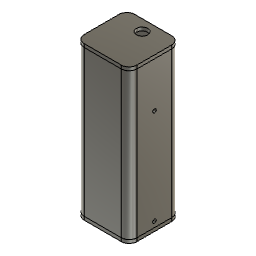
Blinds Device v2 (Autodesk Fusion 360 design; units mm, degrees)
Autodesk Fusion 360 part; units mm, degrees
sketch "Sketch1" plane through (0, 0, 0) normal (0, 0, 1) x (1, 0, 0)
  line L0 (0, 0) -> (39, 0)
  line L1 (0, 0) -> (0, 39)
  line L2 (0, 39) -> (39, 39)
  line L3 (39, 39) -> (39, 0)
  line L4 (39, 0) -> (0, 0)
  line L5 (0, 0) -> (0, 39)
  line L6 (0, 0) -> (3, 0)
  line L7 (39, 39) -> (36, 39)
  line L8 (39, 39) -> (42, 39)
  line L9 (0, 0) -> (-3, 0)
  line L10 (42, 39) -> (42, 42)
  line L11 (-3, 0) -> (-3, -3)
  line L12 (-3, -3) -> (42, -3)
  line L13 (42, -3) -> (42, 42)
  line L14 (42, 42) -> (-3, 42)
  line L15 (-3, 42) -> (-3, -3)
  dimension "d2" = 39
  dimension "d7" = 3
  dimension "d8" = 3
  dimension "d9" = 3
  dimension "d10" = 3
  constraint coincident L0.start L1.start
  constraint horizontal L0
  constraint vertical L1
  constraint horizontal L2
  constraint vertical L3
  constraint horizontal L4
  constraint vertical L5
  constraint perpendicular L1 L6
  constraint perpendicular L3 L7
  constraint perpendicular L3 L8
  constraint perpendicular L1 L9
  constraint perpendicular L8 L10
  constraint perpendicular L9 L11
  constraint horizontal L12
  constraint vertical L13
  constraint horizontal L14
  constraint vertical L15
  measures "d2" distance of L0.start L1.end
  measures "d7" distance of L2.end L8.end
  measures "d8" distance of L0.start L9.end
  measures "d9" distance of L8.end L10.end
  measures "d10" distance of L9.end L11.end
extrude "Extrude1" add sketch "Sketch1" along normal blind 130 contours L1 L2 L5 L7 L8 L9 L10 L13 L14 L15 | L0 L3 L4 L6 L8 L9 L11 L12 L13 L15 makes body 1
sketch "Sketch2" plane through (0, 0, 130) normal (0, 0, 1) x (-1, 0, 0)
  line L0 (-39, -39) -> (-39, 0)
  line L1 (-39, 0) -> (0, 0)
  line L2 (0, 0) -> (0, -39)
  line L3 (0, -39) -> (-39, -39)
  line L4 (3, -42) -> (3, 3)
  line L5 (3, 3) -> (-42, 3)
  line L6 (-42, 3) -> (-42, -42)
  line L7 (-42, -42) -> (3, -42)
  line L8 (3, -42) -> (-42, -42)
  line L9 (-42, -42) -> (-42, 3)
  line L10 (-42, 3) -> (3, 3)
  line L11 (3, 3) -> (3, -42)
  line L12 (-19.5, -42) -> (-19.5, -32)
  circle A0 centre (-19.5, -32) radius 5
  dimension "d13" = 10
  dimension "d14" = 10
  constraint horizontal L8
  constraint vertical L9
  constraint horizontal L10
  constraint vertical L11
  constraint coincident L5.end L6.start
  constraint coincident L4.start L7.end
  constraint midpoint L8 L12.start
  constraint perpendicular L8 L12
  constraint coincident L12.end A0.centre
  measures "d13" distance of L12.start L12.end
  measures "d14" diameter of A0
extrude "Extrude2" add sketch "Sketch2" along normal blind 3 separate body contours L0 L1 L2 L3 | L4 L5 L6 L7 L8 L9 L10 L11 makes body 2
extrude "Extrude3" cut 1 faces at (39, 26, 86.6667) along direction (1, 0, 0) blind 1 on bodies 1 bodies 1
extrude "Extrude4" cut 1 faces at (0, 13, 86.6667) along direction (-1, 0, 0) blind 1 on bodies 1 bodies 1
extrude "Extrude5" cut 1 faces at (-1, 13, 86.6667) along direction (-1, 0, 0) blind 1 on bodies 1 bodies 1
extrude "Extrude6" cut 1 faces at (40, 26, 86.6667) along direction (1, 0, 0) blind 1 on bodies 1 bodies 1
extrude "Extrude7" add 1 faces at (42, 12, 86.6667) along direction (1, 0, 0) blind 1 on bodies 1 bodies 1
extrude "Extrude8" add 1 faces at (-3, 27, 86.6667) along direction (-1, 0, 0) blind 1 on bodies 1 bodies 1
extrude "Extrude9" add 1 faces at (-3, 27, 132) along direction (-1, 0, 0) blind 1 on bodies 2 bodies 2
extrude "Extrude10" add 1 faces at (42, 12, 132) along direction (1, 0, 0) blind 1 on bodies 2 bodies 2
sketch "Sketch3" plane through (0, 0, 130) normal (0, 0, -1) x (1, 0, 0)
  circle A0 centre (19.5, -32) radius 5
  line L0 (43, 3) -> (-4, 3)
  line L1 (-4, 3) -> (-4, -42)
  line L2 (-4, -42) -> (43, -42)
  line L3 (43, -42) -> (43, 3)
  line L4 (43, 3) -> (40.8, 3)
  line L5 (40.8, 3) -> (40.8, -42)
  line L6 (19.5, -42) -> (19.5, 3)
  line L7 (43, -19.5) -> (-4, -19.5)
  line L8 (40.8, 3) -> (40.8, -0.2)
  line L9 (40.8, -0.2) -> (38.8, -0.2)
  line L10 (38.8, -0.2) -> (40.8, -0.2)
  line L11 (40.8, -0.2) -> (40.8, -10.2)
  line L12 (40.8, -10.2) -> (38.8, -10.2)
  line L13 (38.8, -10.2) -> (38.8, -0.2)
  line L14 (38.8, -28.8) -> (38.8, -38.8)
  line L15 (38.8, -38.8) -> (40.8, -38.8)
  line L16 (40.8, -28.8) -> (38.8, -28.8)
  line L17 (40.8, -38.8) -> (40.8, -28.8)
  line L18 (-1.8, -38.8) -> (-1.8, -28.8)
  line L19 (-1.8, -28.8) -> (0.2, -28.8)
  line L20 (0.2, -28.8) -> (0.2, -38.8)
  line L21 (0.2, -38.8) -> (-1.8, -38.8)
  line L22 (-1.8, -0.2) -> (-1.8, -10.2)
  line L23 (-1.8, -10.2) -> (0.2, -10.2)
  line L24 (-1.8, -0.2) -> (0.2, -0.2)
  line L25 (0.2, -10.2) -> (0.2, -0.2)
  dimension "d33" = 2.2
  dimension "d34" = 3.2
  dimension "d35" = 2
  dimension "d36" = 10
  constraint coincident L0.start L3.end
  constraint perpendicular L3 L4
  constraint coincident L2 L5.end
  constraint perpendicular L2 L5
  constraint midpoint L2 L6.start
  constraint midpoint L0 L6.end
  constraint midpoint L3 L7.start
  constraint midpoint L1 L7.end
  constraint perpendicular L4 L8
  constraint perpendicular L8 L9
  constraint horizontal L10
  constraint vertical L11
  constraint horizontal L12
  constraint vertical L13
  constraint symmetric L7 L9.end L14.end
  constraint symmetric L7 L8.end L15.end
  constraint symmetric L7 L11.end L16.start
  constraint symmetric L7 L12.end L14.start
  constraint symmetric L6 L8.end L22.start
  constraint symmetric L6 L9.end L24.end
  constraint symmetric L6 L11.end L22.end
  constraint symmetric L6 L12.end L23.end
  constraint symmetric L6 L14.start L19.end
  constraint symmetric L6 L14.end L20.end
  constraint symmetric L6 L15.end L18.start
  constraint symmetric L6 L16.start L18.end
  measures "d33" distance of L0.start L4.end
  measures "d34" distance of L4.end L8.end
  measures "d35" distance of L8.end L9.end
  measures "d36" distance of L9.end L12.end
extrude "Extrude11" add sketch "Sketch3" along normal blind 10 contours L5 L9 L10 L11 L12 L13 | L5 L14 L15 L16 L17 | L18 L19 L20 L21 | L22 L23 L24 L25 bodies 2
copy_body "CopyPasteBodies1" bodies 2 makes body 3
move_body "Move1" bodies 3 to x (1, 0, 0) y (0, -1, 0) z (0, 0, -1) at (0, -6, 100)
move_body "Move2" bodies 3 to x (1, 0, 0) y (0, 1, 0) z (0, 0, 1) at (0, 45, 30)
move_face "OffsetFaces1" offset 6 1 faces at (14.5248, 7.4978, -1) on bodies 3
sketch "Sketch4" plane through (0, 0, -3) normal (0, 0, -1) x (1, 0, 0)
  line L0 (-4, -42) -> (43, -42)
  line L1 (43, -42) -> (43, 3)
  line L2 (43, 3) -> (-4, 3)
  line L3 (-4, 3) -> (-4, -42)
  line L4 (19.5, 3) -> (19.5, -42)
  line L5 (43, -19.5) -> (-4, -19.5)
  circle A0 centre (19.5, -19.5) radius 2.5
  dimension "d40" = 5
  constraint midpoint L2 L4.start
  constraint midpoint L0 L4.end
  constraint midpoint L1 L5.start
  constraint midpoint L3 L5.end
  constraint midpoint L4 A0.centre
  measures "d40" diameter of A0
extrude "Extrude12" cut sketch "Sketch4" against normal blind 3 contours L4 L5 A0 | L4 L5 A0 | L4 L5 A0 | L4 L5 A0 bodies 3
fillet "Fillet1" radius 7 12 edges at (43, 42, 65) (43, -3, 65) (-4, 42, 65) (-4, -3, 65) (43, 42, 131.5) (43, -3, 131.5) (-4, 42, 131.5) (-4, -3, 131.5) (43, -3, -1.5) (43, 42, -1.5) (-4, 42, -1.5) (-4, -3, -1.5) on bodies 1 2 3
sketch "Sketch5" plane through (-4, 0, 0) normal (-1, 0, 0) x (0, -1, 0)
  line L0 (-4, 0) -> (-4, 130)
  line L1 (-4, 130) -> (-35, 130)
  line L2 (-35, 130) -> (-35, 0)
  line L3 (-35, 0) -> (-4, 0)
  line L4 (-19.5, 130) -> (-19.5, 90)
  circle A0 centre (-19.5, 90) radius 1.6
  dimension "d45" = 40
  dimension "d46" = 3.2
  constraint midpoint L1 L4.start
  constraint perpendicular L1 L4
  constraint coincident L4.end A0.centre
  measures "d45" distance of L4.start L4.end
  measures "d46" diameter of A0
extrude "Extrude13" cut sketch "Sketch5" against normal blind 50 contours A0 bodies 1
extrude "Extrude14" cut 4 faces at (39.4667, 35.4667, 10) (39.4667, 6.8667, 10) (-0.4667, 35.4667, 10) (-1.1333, 6.8667, 10) along direction (0, 0, -1) blind 10 on bodies 3 bodies 3
sketch "Sketch6" plane through (0, 0, 0) normal (0, 0, 1) x (-1, 0, 0)
  arc A0 (4, -4) -> (-3, 3) centre (-3, -4) ccw
  line L0 (-3, 3) -> (-36, 3)
  arc A1 (-36, 3) -> (-43, -4) centre (-36, -4) ccw
  line L1 (-43, -4) -> (-43, -35)
  arc A2 (-43, -35) -> (-36, -42) centre (-36, -35) ccw
  line L2 (-36, -42) -> (-3, -42)
  arc A3 (-3, -42) -> (4, -35) centre (-3, -35) ccw
  line L3 (4, -35) -> (4, -4)
  circle A4 centre (-19.5, -19.5) radius 2.5
  line L4 (4, -19.5) -> (1.8, -19.5)
  line L5 (-19.5, -42) -> (-19.5, 3)
  line L6 (1.8, -19.5) -> (1.8, -9.5)
  line L7 (1.8, -19.5) -> (1.8, -29.5)
  line L8 (1.8, -29.5) -> (-1.2, -29.5)
  line L9 (-1.2, -29.5) -> (1.8, -29.5)
  line L10 (1.8, -29.5) -> (1.8, -9.5)
  line L11 (1.8, -9.5) -> (-1.2, -9.5)
  line L12 (-1.2, -9.5) -> (-1.2, -29.5)
  line L13 (-37.8, -9.5) -> (-37.8, -29.5)
  line L14 (-40.8, -9.5) -> (-37.8, -9.5)
  line L15 (-40.8, -29.5) -> (-40.8, -9.5)
  line L16 (-40.8, -29.5) -> (-37.8, -29.5)
  dimension "d51" = 2.2
  dimension "d52" = 45
  dimension "d53" = 10
  dimension "d54" = 10
  dimension "d55" = 3
  constraint midpoint L3 L4.start
  constraint perpendicular L3 L4
  constraint midpoint L2 L5.start
  constraint midpoint L0 L5.end
  constraint perpendicular L4 L6
  constraint perpendicular L4 L7
  constraint perpendicular L7 L8
  constraint horizontal L9
  constraint vertical L10
  constraint horizontal L11
  constraint vertical L12
  constraint symmetric L5 L6.end L14.start
  constraint symmetric L5 L7.end L15.start
  constraint symmetric L5 L8.end L13.end
  constraint symmetric L5 L11.end L13.start
  measures "d51" distance of L4.start L4.end
  measures "d52" distance of L5.start L5.end
  measures "d53" distance of L4.end L6.end
  measures "d54" distance of L4.end L7.end
  measures "d55" distance of L7.end L8.end
extrude "Extrude15" add sketch "Sketch6" along normal blind 10 contours L6 L7 L8 L9 L10 L11 L12 | L13 L14 L15 L16 bodies 3
sketch "Sketch7" plane through (-1.8, 0, 0) normal (-1, 0, 0) x (0, -1, 0)
  line L0 (-29.5, 0) -> (-9.5, 0)
  line L1 (-9.5, 0) -> (-9.5, 10)
  line L2 (-9.5, 10) -> (-29.5, 10)
  line L3 (-29.5, 10) -> (-29.5, 0)
  line L4 (-29.5, 5) -> (-9.5, 5)
  circle A0 centre (-19.5, 5) radius 1.6
  dimension "d58" = 20
  dimension "d59" = 3.2
  constraint midpoint L3 L4.start
  constraint midpoint L1 L4.end
  constraint midpoint L4 A0.centre
  measures "d58" distance of L4.start L4.end
  measures "d59" diameter of A0
extrude "Extrude16" cut sketch "Sketch7" along normal blind 20 and the other way blind 58 contours L4 A0 | L4 A0 bodies 1 3
named bodies: "main", "top", "bottom"
